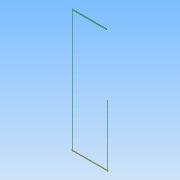
# Autodesk Inventor part: BAO Text
Saved by Autodesk Inventor 2013 (Build 170138000, 138)
## iProperties
Created: 2018-08-01
Part Number: BAO Text
Material: Generic
Document SubType Name: Modeling
Designer: Jeff Vyduna
Density: 1 g/cm^3
Author: Jeff Vyduna
Autodesk Inventor part; units mm, degrees
ref_plane "YZ Plane" through (0, 0, 0) normal (1, 0, 0) x (0, 1, 0)
ref_plane "XZ Plane" through (0, 0, 0) normal (0, 1, 0) x (-1, 0, 0)
ref_plane "XY Plane" through (0, 0, 0) normal (0, 0, 1) x (1, 0, 0)
ref_plane "Work Plane1" through (0, 0, 0) normal (0, 0, 1) x (1, 0, 0)
sketch "Sketch1" plane through (0, 0, 0) normal (0, 0, 1) x (1, 0, 0)
  line L0 (-277.0188, -19.05) -> (-277.0187, 958.85)
  line L1 (264.3188, 1911.35) -> (-264.3187, 1911.35)
  line L2 (-277.0187, 958.85) -> (-277.0187, 1936.75)
  line L3 (-264.3187, 1924.05) -> (264.3188, 1924.05)
  line L4 (277.0187, 958.85) -> (277.0187, -19.05)
  line L5 (264.3188, -6.35) -> (-264.3188, -6.35)
  line L6 (277.0188, 1936.75) -> (277.0187, 958.85)
  line L7 (-277.0188, -6.35) -> (277.0187, -6.35)
  line L8 (277.0187, 958.85) -> (274.6375, 1924.05)
  line L9 (274.6375, 1924.05) -> (-274.6375, 1924.05)
  line L10 (-274.6375, 1924.05) -> (-277.0187, 958.85)
  point P0 (0, 0)
extrude "Extrusion1" add sketch "Sketch1" along normal blind 5.588
sketch "Sketch2" plane through (0, 0, 5.588) normal (0, 0, 1) x (1, 0, 0)
  line L0 (277.0187, -6.35) -> (277.0187, 958.85) projected
  line L1 (-274.6375, 1924.05) -> (277.0187, 1924.05) construction
  line L2 (277.0187, 1924.05) -> (277.0187, 0) construction
  line L3 (277.0187, 0) -> (-274.6375, 0) construction
  line L4 (-274.6375, 0) -> (-274.6375, 1924.05) construction
  spline S0 degree 2 poles (165.4568, 2131.2708) (187.75, 2161.3863) (187.75, 2195.8039) knots 0 0 0 1 1 1
  spline S1 degree 2 poles (187.75, 2195.8039) (187.75, 2229.8305) (151.7679, 2288.497) (91.1459, 2322.9147) (55.946, 2322.9147) knots 0 0 0 1 2 3 3 3
  line L5 (55.946, 2322.9147) -> (-179.111, 2322.9147)
  line L6 (-179.111, 2322.9147) -> (-179.111, 1924.7648)
  line L7 (-179.111, 1924.7648) -> (-197.1021, 1924.7648)
  line L8 (-197.1021, 1924.7648) -> (-197.1021, 2340.9057)
  line L9 (-197.1021, 2340.9057) -> (55.946, 2340.9057)
  spline S2 degree 2 poles (55.946, 2340.9057) (95.8392, 2340.9057) (165.0657, 2301.7947) (205.7411, 2234.5238) (205.7411, 2195.8039) knots 0 0 0 1 2 3 3 3
  spline S3 degree 2 poles (205.7411, 2195.8039) (205.7411, 2159.0396) (185.0123, 2131.2708) knots 0 0 0 1 1 1
  spline S4 degree 2 poles (185.0123, 2131.2708) (205.7411, 2102.3287) (205.7411, 2072.2132) knots 0 0 0 1 1 1
  spline S5 degree 2 poles (205.7411, 2072.2132) (205.7411, 2038.5778) (181.8834, 1982.6491) (140.8168, 1945.4936) (86.4526, 1924.7648) (55.946, 1924.7648) knots 0 0 0 1 2 3 4 4 4
  line L10 (55.946, 1924.7648) -> (-60.6047, 1924.7648)
  line L11 (-60.6047, 1924.7648) -> (-60.6047, 1942.7559)
  line L12 (-60.6047, 1942.7559) -> (55.946, 1942.7559)
  spline S6 degree 2 poles (55.946, 1942.7559) (82.5415, 1942.7559) (130.648, 1962.7025) (166.6301, 1996.729) (187.75, 2045.2266) (187.75, 2072.2132) knots 0 0 0 1 2 3 4 4 4
  spline S7 degree 2 poles (187.75, 2072.2132) (187.75, 2084.3376) (176.4078, 2118.3642) (165.4568, 2131.2708) knots 0 0 0 1 2 2 2
  spline S8 degree 2 poles (169.759, 2195.8039) (169.759, 2160.6041) (144.7279, 2132.4441) knots 0 0 0 1 1 1
  spline S9 degree 2 poles (144.7279, 2132.4441) (169.759, 2104.6753) (169.759, 2072.2132) knots 0 0 0 1 1 1
  spline S10 degree 2 poles (169.759, 2072.2132) (169.759, 2040.9244) (138.4702, 1989.2979) (86.4526, 1961.138) (55.946, 1961.138) knots 0 0 0 1 2 3 3 3
  line L13 (55.946, 1961.138) -> (-60.6047, 1961.138)
  line L14 (-60.6047, 1961.138) -> (-60.6047, 1979.1291)
  line L15 (-60.6047, 1979.1291) -> (55.946, 1979.1291)
  spline S11 degree 2 poles (55.946, 1979.1291) (95.4481, 1979.1291) (151.7679, 2031.5378) (151.7679, 2072.2132) knots 0 0 0 1 2 2 2
  spline S12 degree 2 poles (151.7679, 2072.2132) (151.7679, 2086.6843) (136.9057, 2122.2753) (123.608, 2131.6619) knots 0 0 0 1 2 2 2
  spline S13 degree 2 poles (123.608, 2131.6619) (151.7679, 2157.8663) (151.7679, 2195.8039) knots 0 0 0 1 1 1
  spline S14 degree 2 poles (151.7679, 2195.8039) (151.7679, 2232.5683) (94.2748, 2286.5414) (55.946, 2286.5414) knots 0 0 0 1 2 2 2
  line L16 (55.946, 2286.5414) -> (-142.7378, 2286.5414)
  line L17 (-142.7378, 2286.5414) -> (-142.7378, 1924.7648)
  line L18 (-142.7378, 1924.7648) -> (-161.12, 1924.7648)
  line L19 (-161.12, 1924.7648) -> (-161.12, 2304.9236)
  line L20 (-161.12, 2304.9236) -> (55.946, 2304.9236)
  spline S15 degree 2 poles (55.946, 2304.9236) (86.0615, 2304.9236) (138.4702, 2275.1992) (169.759, 2224.7461) (169.759, 2195.8039) knots 0 0 0 1 2 3 3 3
  line L21 (-60.6047, 2138.7019) -> (55.946, 2138.7019)
  spline S16 degree 2 poles (55.946, 2138.7019) (80.977, 2138.7019) (115.3947, 2168.8174) (115.3947, 2195.8039) knots 0 0 0 1 2 2 2
  spline S17 degree 2 poles (115.3947, 2195.8039) (115.3947, 2217.7061) (79.4126, 2250.5593) (55.946, 2250.5593) knots 0 0 0 1 2 2 2
  line L22 (55.946, 2250.5593) -> (-106.7557, 2250.5593)
  line L23 (-106.7557, 2250.5593) -> (-106.7557, 1924.7648)
  line L24 (-106.7557, 1924.7648) -> (-124.7468, 1924.7648)
  line L25 (-124.7468, 1924.7648) -> (-124.7468, 2268.5504)
  line L26 (-124.7468, 2268.5504) -> (55.946, 2268.5504)
  spline S18 degree 2 poles (55.946, 2268.5504) (87.2348, 2268.5504) (133.3858, 2225.1372) (133.3858, 2195.8039) knots 0 0 0 1 2 2 2
  spline S19 degree 2 poles (133.3858, 2195.8039) (133.3858, 2173.1196) (112.2658, 2138.7019) (94.2748, 2129.7064) knots 0 0 0 1 2 2 2
  spline S20 degree 2 poles (94.2748, 2129.7064) (133.3858, 2115.6264) (133.3858, 2072.2132) knots 0 0 0 1 1 1
  spline S21 degree 2 poles (133.3858, 2072.2132) (133.3858, 2038.1867) (88.4081, 1997.1201) (55.946, 1997.1201) knots 0 0 0 1 2 2 2
  line L27 (55.946, 1997.1201) -> (-60.6047, 1997.1201)
  line L28 (-60.6047, 1997.1201) -> (-60.6047, 2015.1112)
  line L29 (-60.6047, 2015.1112) -> (55.946, 2015.1112)
  spline S22 degree 2 poles (55.946, 2015.1112) (80.977, 2015.1112) (115.3947, 2045.2266) (115.3947, 2072.2132) knots 0 0 0 1 2 2 2
  spline S23 degree 2 poles (115.3947, 2072.2132) (115.3947, 2090.5954) (89.1903, 2118.7553) (63.7682, 2121.102) knots 0 0 0 1 2 2 2
  spline S24 degree 2 poles (63.7682, 2121.102) (61.4215, 2120.7108) (55.946, 2120.7108) knots 0 0 0 1 1 1
  line L30 (55.946, 2120.7108) -> (-60.6047, 2120.7108)
  line L31 (-60.6047, 2120.7108) -> (-60.6047, 2138.7019)
  line L32 (-70.3825, 1924.7648) -> (-88.7646, 1924.7648)
  line L33 (-88.7646, 1924.7648) -> (-88.7646, 2232.5683)
  line L34 (-88.7646, 2232.5683) -> (55.946, 2232.5683)
  spline S25 degree 2 poles (55.946, 2232.5683) (73.1548, 2232.5683) (97.4036, 2211.4483) (97.4036, 2195.8039) knots 0 0 0 1 2 2 2
  spline S26 degree 2 poles (97.4036, 2195.8039) (97.4036, 2175.4662) (74.7193, 2157.0841) (55.946, 2157.0841) knots 0 0 0 1 2 2 2
  line L35 (55.946, 2157.0841) -> (-60.6047, 2157.0841)
  line L36 (-60.6047, 2157.0841) -> (-60.6047, 2175.0751)
  line L37 (-60.6047, 2175.0751) -> (55.946, 2175.0751)
  spline S27 degree 2 poles (55.946, 2175.0751) (79.4126, 2175.0751) (79.4126, 2195.8039) knots 0 0 0 1 1 1
  spline S28 degree 2 poles (79.4126, 2195.8039) (79.4126, 2204.4084) (66.1149, 2214.1861) (55.946, 2214.1861) knots 0 0 0 1 2 2 2
  line L38 (55.946, 2214.1861) -> (-70.3825, 2214.1861)
  line L39 (-70.3825, 2214.1861) -> (-70.3825, 1924.7648)
  spline S29 degree 2 poles (79.4126, 2069.8666) (79.4126, 2079.6443) (67.2882, 2086.2932) (55.946, 2086.2932) knots 0 0 0 1 2 2 2
  line L40 (55.946, 2086.2932) -> (-60.6047, 2086.2932)
  line L41 (-60.6047, 2086.2932) -> (-60.6047, 2104.2842)
  line L42 (-60.6047, 2104.2842) -> (55.946, 2104.2842)
  spline S30 degree 2 poles (55.946, 2104.2842) (97.4036, 2104.2842) (97.4036, 2069.8666) knots 0 0 0 1 1 1
  spline S31 degree 2 poles (97.4036, 2069.8666) (97.4036, 2050.3111) (74.7193, 2033.4933) (55.946, 2033.4933) knots 0 0 0 1 2 2 2
  line L43 (55.946, 2033.4933) -> (-60.6047, 2033.4933)
  line L44 (-60.6047, 2033.4933) -> (-60.6047, 2051.4844)
  line L45 (-60.6047, 2051.4844) -> (55.946, 2051.4844)
  spline S32 degree 2 poles (55.946, 2051.4844) (79.4126, 2051.4844) (79.4126, 2069.8666) knots 0 0 0 1 1 1
  line L46 (-211.9643, 762.9501) -> (-231.5198, 762.9501)
  line L47 (-231.5198, 762.9501) -> (-66.8625, 1179.091)
  line L48 (-66.8625, 1179.091) -> (-47.307, 1179.091)
  line L49 (-47.307, 1179.091) -> (116.9591, 762.9501)
  line L50 (116.9591, 762.9501) -> (97.7948, 762.9501)
  line L51 (97.7948, 762.9501) -> (-57.0848, 1154.8422)
  line L52 (-57.0848, 1154.8422) -> (-211.9643, 762.9501)
  line L53 (30.5239, 1179.091) -> (195.1811, 762.9501)
  line L54 (195.1811, 762.9501) -> (175.6256, 762.9501)
  line L55 (175.6256, 762.9501) -> (10.9684, 1179.091)
  line L56 (10.9684, 1179.091) -> (30.5239, 1179.091)
  line L57 (-8.5871, 1179.091) -> (156.0701, 762.9501)
  line L58 (156.0701, 762.9501) -> (136.5146, 762.9501)
  line L59 (136.5146, 762.9501) -> (-27.7515, 1179.091)
  line L60 (-27.7515, 1179.091) -> (-8.5871, 1179.091)
  line L61 (233.901, 762.9501) -> (214.3455, 762.9501)
  line L62 (214.3455, 762.9501) -> (50.0793, 1179.091)
  line L63 (50.0793, 1179.091) -> (69.2437, 1179.091)
  line L64 (69.2437, 1179.091) -> (233.901, 762.9501)
  line L65 (-54.7381, 1111.8201) -> (-44.5692, 1088.7446)
  line L66 (-44.5692, 1088.7446) -> (-173.2444, 762.9501)
  line L67 (-173.2444, 762.9501) -> (-192.4088, 762.9501)
  line L68 (-192.4088, 762.9501) -> (-54.7381, 1111.8201)
  line L69 (-34.7915, 1064.1047) -> (-25.0137, 1039.0736)
  line L70 (-25.0137, 1039.0736) -> (-133.7423, 762.9501)
  line L71 (-133.7423, 762.9501) -> (-153.6889, 762.9501)
  line L72 (-153.6889, 762.9501) -> (-34.7915, 1064.1047)
  line L73 (-15.6271, 1014.4337) -> (-5.8494, 989.0116)
  line L74 (-5.8494, 989.0116) -> (-95.4135, 762.9501)
  line L75 (-95.4135, 762.9501) -> (-114.5779, 762.9501)
  line L76 (-114.5779, 762.9501) -> (-15.6271, 1014.4337)
  line L77 (-64.907, 812.621) -> (-57.867, 831.0032)
  line L78 (-57.867, 831.0032) -> (61.0304, 831.0032)
  line L79 (61.0304, 831.0032) -> (68.4615, 812.621)
  line L80 (68.4615, 812.621) -> (-64.907, 812.621)
  line L81 (-50.827, 848.9942) -> (-43.787, 866.9853)
  line L82 (-43.787, 866.9853) -> (46.5594, 866.9853)
  line L83 (46.5594, 866.9853) -> (54.3816, 848.9942)
  line L84 (54.3816, 848.9942) -> (-50.827, 848.9942)
  line L85 (-36.747, 884.9764) -> (-29.316, 903.3585)
  line L86 (-29.316, 903.3585) -> (32.4794, 903.3585)
  line L87 (32.4794, 903.3585) -> (39.9105, 884.9764)
  line L88 (39.9105, 884.9764) -> (-36.747, 884.9764)
  spline S33 degree 2 poles (-206.8798, -278.7939) (-224.8709, -236.9452) (-224.8709, -144.6432) (-188.8888, -60.9457) (-128.2668, -0.7148) (-44.5692, 35.2673) (47.3416, 35.2673) (131.0391, -0.7148) (191.6611, -60.9457) (227.6432, -144.6432) (227.6432, -236.9452) (191.6611, -320.6427) (131.0391, -380.8736) (47.3416, -416.8557) (-44.5692, -416.8557) (-128.2668, -380.8736) (-188.8888, -320.6427) (-206.8798, -278.7939) knots 0 0 0 1 2 3 4 5 6 7 8 9 10 11 12 13 14 15 16 16 16
  spline S34 degree 2 poles (-190.4532, -109.8345) (-206.8798, -148.5543) (-206.8798, -233.0341) (-174.0266, -310.0827) (-118.0979, -366.0114) (-41.0492, -398.8647) (43.4305, -398.8647) (120.8702, -366.0114) (176.4078, -310.0827) (209.2611, -233.0341) (209.2611, -148.5543) (176.4078, -71.5057) (120.8702, -15.577) (43.4305, 17.2762) (-41.0492, 17.2762) (-118.0979, -15.577) (-174.0266, -71.5057) (-190.4532, -109.8345) knots 0 0 0 1 2 3 4 5 6 7 8 9 10 11 12 13 14 15 16 16 16
  spline S35 degree 2 poles (-163.0755, -285.8339) (-188.4977, -242.4207) (-188.4977, -139.1677) (-137.6534, -51.9502) (-50.0448, -0.7148) (52.8171, -0.7148) (140.4257, -51.9502) (191.27, -139.1677) (191.27, -242.4207) (140.4257, -329.6382) (52.8171, -380.8736) (-50.0448, -380.8736) (-137.6534, -329.6382) (-163.0755, -285.8339) knots 0 0 0 1 2 3 4 5 6 7 8 9 10 11 12 12 12
  spline S36 degree 2 poles (-157.2089, -123.9144) (-170.5066, -155.9854) (-170.5066, -225.603) (-143.52, -289.3539) (-97.3691, -335.5049) (-33.6182, -362.4914) (36.3905, -362.4914) (100.1414, -335.5049) (145.9013, -289.3539) (173.279, -225.603) (173.279, -155.9854) (145.9013, -91.8434) (100.1414, -46.0835) (36.3905, -18.7059) (-33.6182, -18.7059) (-97.3691, -46.0835) (-143.52, -91.8434) (-157.2089, -123.9144) knots 0 0 0 1 2 3 4 5 6 7 8 9 10 11 12 13 14 15 16 16 16
  spline S37 degree 2 poles (-131.7867, -267.8428) (-152.5156, -232.643) (-152.5156, -148.9454) (-111.449, -78.1546) (-40.267, -37.088) (43.0394, -37.088) (113.8303, -78.1546) (155.2879, -148.9454) (155.2879, -232.643) (113.8303, -303.4338) (43.0394, -344.5004) (-40.267, -344.5004) (-111.449, -303.4338) (-131.7867, -267.8428) knots 0 0 0 1 2 3 4 5 6 7 8 9 10 11 12 12 12
  spline S38 degree 2 poles (-116.1423, -122.7411) (-134.5245, -153.6388) (-134.5245, -227.5585) (-98.1513, -290.1361) (-35.5737, -326.5093) (38.3461, -326.5093) (100.5325, -290.1361) (136.9057, -227.5585) (136.9057, -153.6388) (100.5325, -91.4523) (38.3461, -55.0791) (-35.5737, -55.0791) (-98.1513, -91.4523) (-116.1423, -122.7411) knots 0 0 0 1 2 3 4 5 6 7 8 9 10 11 12 12 12
  spline S39 degree 2 poles (-107.1468, -236.5541) (-116.1423, -214.6519) (-116.1423, -166.9365) (-97.7602, -123.5233) (-66.0803, -91.8434) (-22.6671, -73.0701) (25.0483, -73.0701) (68.8526, -91.8434) (100.1414, -123.5233) (118.9147, -166.9365) (118.9147, -214.6519) (100.1414, -258.0651) (68.8526, -289.745) (25.0483, -308.5183) (-22.6671, -308.5183) (-66.0803, -289.745) (-97.7602, -258.0651) (-107.1468, -236.5541) knots 0 0 0 1 2 3 4 5 6 7 8 9 10 11 12 13 14 15 16 16 16
  spline S40 degree 2 poles (-69.2092, -120.3944) (-98.1513, -149.7277) (-98.1513, -231.8607) (-39.8759, -290.1361) (42.6483, -290.1361) (100.9236, -231.8607) (100.9236, -149.7277) (42.6483, -91.0612) (-39.8759, -91.0612) (-69.2092, -120.3944) knots 0 0 0 1 2 3 4 5 6 7 8 8 8
  point P0 (0, 0)
  constraints: 1 point on line, 2 other
extrude "Extrusion2" add sketch "Sketch2" along normal blind 25.4
equation "\"d1\" = d0"
equation "\"d0\" = 2.38125"
body "Solid1"
